Autodesk Inventor part; units mm, degrees
note: some values were not read from the file. Chosen so that the rebuilt part matches the saved one: direction of "Hole2".
(part 20 of 20)
sketch "Sketch20" plane through (0, 13.762, -7.5) normal (0, 1, 0) x (-1, 0, 0)
  line L0 (9.984, 11.484) -> (-9.984, 11.484)
  line L1 (-9.984, 11.484) -> (-9.984, -31.460908)
  line L2 (-9.984, -31.460908) -> (9.984, -31.460908)
  line L3 (9.984, -31.460908) -> (9.984, 11.484)
  point P0 (0, 7.5)
  constraints: 8 end point, 2 parallel, 1 coincident, 1 horizontal, 1 perpendicular
loft "Loft1" [suppressed]
sketch "Sketch21" plane through (0, 25.262, -7.5) normal (0, 1, 0) x (1, 0, 0)
  line L0 (12.208699, 33.685607) -> (12.208699, -13.708699)
  line L1 (11, 32.476908) -> (-11, 32.476908)
  line L2 (-12.208699, 33.685607) -> (12.208699, 33.685607)
  line L3 (12.208699, 33.685607) -> (12.208699, 32.844773)
  line L4 (12.208699, 32.844773) -> (-12.208699, 32.844773)
  line L5 (-12.208699, 32.844773) -> (-12.208699, 33.685607)
  point P0 (0, -7.5)
  constraints: 8 end point, 2 parallel, 1 horizontal, 1 perpendicular, 1 point on line
extrude "Extrusion14" [suppressed]
ref_plane "Work Plane11" through (0, 0, -53) normal (0, 0, -1) x (-1, 0, 0)
sketch "Sketch29" plane through (2.947448, 25.262, -39.185607) normal (0, 0.9876883, 0.1564345) x (1, 0, 0)
  line L0 (-19.844177, 3.851731) -> (23.663444, 3.851731)
  line L1 (23.663444, 3.851731) -> (23.663444, -48.231307)
  line L2 (23.663444, -48.231307) -> (-19.844177, -48.231307)
  line L3 (-19.844177, -48.231307) -> (-19.844177, 3.851731)
  point P0 (0, 0)
  constraints: 8 end point, 2 parallel, 1 horizontal, 1 perpendicular
extrude "Extrusion16" [suppressed]
sketch "Sketch31" plane through (2.947448, 25.262, -39.185607) normal (0, 0.9876883, 0.1564345) x (1, 0, 0)
  line L0 (8.517951, -45.207586) -> (-14.412847, -45.207586)
  line L1 (-14.412847, -45.207586) -> (-15.156147, 0)
  line L2 (-13.663273, 0.959377) -> (7.663273, 0.959377)
  line L3 (7.663273, 0.959377) -> (7.663273, -44.445586)
  line L4 (7.663273, -44.445586) -> (-13.663273, -44.445586)
  line L5 (-13.663273, -44.445586) -> (-13.663273, 0.959377)
  line L6 (-2.947448, 132.683327) -> (-2.947448, -156.790171)
  line L7 (-13.632147, 0) -> (7.632147, 0)
  line L8 (-15.156147, 1.975377) -> (9.261251, 1.975377)
  point P0 (-2.947448, -42.655014)
  point P1 (-3, 0.959377)
  point P2 (-3, 0)
  dimension "d198" = 1.016
  dimension "d199" = 0.762
  dimension "d200" = 0.762
  constraints: 8 end point, 2 midpoint, 2 parallel, 1 horizontal, 1 perpendicular, 1 vertical alignment
  measures "d198" distance between parallel lines of L2 L8
  measures "d199" distance between parallel lines of L0 L4
  measures "d200" distance from line of L4.end L1
extrude "Extrusion18" [suppressed]
equation "\"d22\" = d24"
equation "\"d23\" = d24"
equation "\"d37\" = t"
equation "\"d40\" = t"
equation "\"t\" = 1.016"
equation "\"d14\" = d24"
equation "\"d24\" = 1.016"
body "Solid1"
